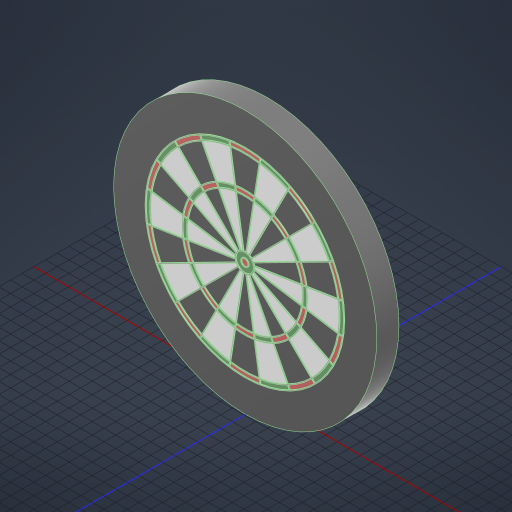
# Autodesk Inventor part: Dartboard
Saved by Autodesk Inventor 2023.2 (Build 272271030, 271C)
## iProperties
Created: 2023-02-20
Part Number: Dartboard
Material: Generisch
Document SubType Name: Modeling
Designer: Stefan
Mass: 6078.2 g
Surface Area: 3858.8 cm^2
Volume: 6078.2 cm^3
Density: 1 g/cm^3
Appearance: Glatt - Waldgrün
Author: Stefan
Autodesk Inventor part; units mm, degrees
ref_plane "YZ Plane" through (0, 0, 0) normal (1, 0, 0) x (0, 1, 0)
ref_plane "XZ Plane" through (0, 0, 0) normal (0, 1, 0) x (-1, 0, 0)
ref_plane "XY Plane" through (0, 0, 0) normal (0, 0, 1) x (1, 0, 0)
sketch "Skizze1" plane through (0, 0, 0) normal (0, 0, 1) x (1, 0, 0)
  circle A0 centre (0, 0) radius 225.45
  circle A1 centre (0, 0) radius 170 construction
  circle A2 centre (0, 0) radius 162 construction
  circle A3 centre (0, 0) radius 107 construction
  circle A4 centre (0, 0) radius 99 construction
  circle A5 centre (0, 0) radius 6.35 construction
  circle A6 centre (0, 0) radius 15.945 construction
  line L0 (0, 225.45) -> (0, -225.45) construction
  line L1 (0, 0) -> (35.2682, 222.6743) construction
  circle A7 centre (0, 0) radius 170.8
  circle A8 centre (0, 0) radius 169.2
  circle A9 centre (0, 0) radius 162.8
  circle A10 centre (0, 0) radius 161.2
  circle A11 centre (0, 0) radius 107.8
  circle A12 centre (0, 0) radius 106.2
  circle A13 centre (0, 0) radius 99.8
  circle A14 centre (0, 0) radius 98.2
  circle A15 centre (0, 0) radius 16.745
  circle A16 centre (0, 0) radius 15.145
  circle A17 centre (0, 0) radius 7.15
  circle A18 centre (0, 0) radius 5.55
  line L2 (25.6783, 167.2401) -> (24.6771, 160.9189)
  line L3 (27.2586, 166.9899) -> (26.2574, 160.6686)
  line L4 (24.4268, 159.3385) -> (16.073, 106.595)
  line L5 (17.6533, 106.3447) -> (26.0071, 159.0883)
  line L6 (14.5712, 97.1129) -> (1.8264, 16.6451)
  line L7 (3.4067, 16.3948) -> (16.1515, 96.8626)
  line L8 (15.8227, 105.0147) -> (14.8215, 98.6933)
  line L9 (17.403, 104.7644) -> (16.4018, 98.443)
  line L10 (-27.2586, 166.9899) -> (-26.2574, 160.6686)
  line L11 (-25.6783, 167.2401) -> (-24.6771, 160.9189)
  line L12 (-26.0071, 159.0883) -> (-17.6533, 106.3447)
  line L13 (-16.073, 106.595) -> (-24.4268, 159.3385)
  line L14 (-17.403, 104.7644) -> (-16.4018, 98.443)
  line L15 (-15.8227, 105.0147) -> (-14.8215, 98.6933)
  line L16 (-16.1515, 96.8626) -> (-3.4067, 16.3948)
  line L17 (-1.8264, 16.6451) -> (-14.5712, 97.1129)
  line L18 (-77.5271, 150.3934) -> (-74.6216, 144.6909)
  line L19 (-76.1015, 151.1198) -> (-73.196, 145.4173)
  line L20 (-73.8952, 143.2653) -> (-49.6516, 95.6847)
  line L21 (-48.226, 96.4111) -> (-72.4696, 143.9917)
  line L22 (-48.9252, 94.259) -> (-46.0196, 88.5564)
  line L23 (-47.4996, 94.9854) -> (-44.594, 89.2828)
  line L24 (-45.2932, 87.1307) -> (-8.3062, 14.5397)
  line L25 (-6.8806, 15.2661) -> (-43.8676, 87.8571)
  point P0 (-3.4067, 16.3948)
  dimension "d1" = 450.9
  dimension "d2" = 340
  dimension "d3" = 8
  dimension "d4" = 8
  dimension "d5" = 12.7
  dimension "d6" = 31.89
  dimension "d7" = 214
  dimension "d8" = 9
  dimension "d10" = 0.8
  dimension "d11" = 1.6
  dimension "d12" = 0.8
  dimension "d13" = 1.6
  dimension "d14" = 0.8
  dimension "d15" = 1.6
  dimension "d16" = 0.8
  dimension "d17" = 1.6
  dimension "d18" = 0.8
  dimension "d19" = 1.6
  dimension "d20" = 0.8
  dimension "d21" = 1.6
  dimension "d22" = 1.6
  dimension "d25" = 36
  constraints: 52 end point, 20 coincident, 19 centre point, 19 point on circle, 6 point on line, 3 parallel, 2 collinear, 1 midpoint, 1 vertical, 53 other
  measures "d1" diameter of A0
  measures "d2" diameter of A1
  measures "d3" radial gap between concentric circles of A2 A1
  measures "d4" radial gap between concentric circles of A4 A3
  measures "d5" diameter of A5
  measures "d6" diameter of A6
  measures "d7" diameter of A3
  measures "d8" angle of L1 L0
  measures "d10" radial gap between concentric circles of A1 A7
  measures "d11" radial gap between concentric circles of A8 A7
  measures "d12" radial gap between concentric circles of A2 A9
  measures "d13" radial gap between concentric circles of A10 A9
  measures "d14" radial gap between concentric circles of A11 A3
  measures "d15" radial gap between concentric circles of A11 A12
  measures "d16" radial gap between concentric circles of A13 A4
  measures "d17" radial gap between concentric circles of A13 A14
  measures "d18" radial gap between concentric circles of A15 A6
  measures "d19" radial gap between concentric circles of A15 A16
  measures "d20" radial gap between concentric circles of A17 A5
  measures "d21" radial gap between concentric circles of A17 A18
  measures "d22" distance between parallel lines of L3 L2
extrude "Extrusion1" add sketch "Skizze1" along normal blind 38 contours L4 A11 L13 A10 | L6 A15 L17 A14
extrude "Extrusion2" add sketch "Skizze1" along normal blind 38 contours L2 A9 L11 A8 | L8 A13 L15 A12
extrude "Extrusion4" add sketch "Skizze1" along normal blind 38 contours A10 L12 A11 L21 | A14 L16 A15 L25
extrude "Extrusion5" add sketch "Skizze1" along normal blind 38 contours A8 L10 A9 L19 | A12 L14 A13 L23
extrude "Extrusion6" add sketch "Skizze1" along normal blind 39 contours L11 A9 L10 A8 | L13 A11 L12 A10 | L15 A13 L14 A12 | L17 A15 L16 A14
extrude "Extrusion7" add sketch "Skizze1" along normal blind 38 contours A16
extrude "Extrusion8" add sketch "Skizze1" along normal blind 38 contours A18
extrude "Extrusion9" add sketch "Skizze1" along normal blind 39 contours A7 | A9 | A11 | A13 | A15 | A17
pattern_circular "Runde Anordnung2" count 10 over 360 about axis through (0, 0, -10) along (0, 0, 1) of "Extrusion1"
pattern_circular "Runde Anordnung3" count 10 over 360 about axis through (0, 0, -10) along (0, 0, 1) of "Extrusion2"
pattern_circular "Runde Anordnung4" count 10 over 360 about axis through (0, 0, -10) along (0, 0, 1) of "Extrusion4"
pattern_circular "Runde Anordnung5" count 10 over 360 about axis through (0, 0, -10) along (0, 0, 1) of "Extrusion5"
pattern_circular "Runde Anordnung6" count 20 over 360 about axis through (0, 0, -10) along (0, 0, 1) of "Extrusion6"
extrude "Extrusion10" add sketch "Skizze1" along normal blind 38 contours A0
